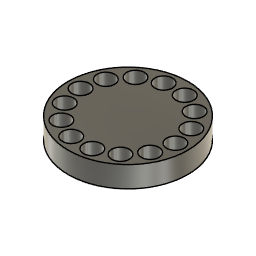
test_roller_pinion v1 (Autodesk Fusion 360 design; units mm, degrees)
Autodesk Fusion 360 part; units mm, degrees
note: some values were not read from the file. Chosen so that the rebuilt part matches the saved one: which face or edge a step refers to.
sketch "Sketch1" plane through (0, 0, 0) normal (0, 0, 1) x (1, 0, 0)
  circle A0 centre (0, 0) radius 17
  line L0 (-17, 0) -> (-16, 0)
  circle A1 centre (-13.5, 0) radius 2.5
  dimension "d1" = 34
  dimension "d2" = 5
  dimension "d7" = 1
  constraint coincident A0.centre origin
  constraint coincident A0 L0.start
  constraint horizontal L0
  constraint coincident L0.end A1
  measures "d1" diameter of A0
  measures "d2" diameter of A1
  measures "d7" distance of L0.start L0.end
extrude "Extrude1" add sketch "Sketch1" along normal blind 6
pattern_circular "C-Pattern1" count 14 over 360 about axis through (0, 0, 6) along (0, 0, 1) of 2 faces at (-15.9676, 0.401, 4) (-11.0081, -0.2012, 4)
sketch "Sketch2" plane through (0, 0, 6) normal (0, 0, 1) x (-1, 0, 0)
  circle A0 centre (-13.5, 0) radius 2.5
  circle A1 centre (-12.1631, 5.8574) radius 2.5
  circle A2 centre (-8.4171, 10.5547) radius 2.5
  circle A3 centre (-3.004, 13.1615) radius 2.5
  circle A4 centre (3.004, 13.1615) radius 2.5
  circle A5 centre (8.4171, 10.5547) radius 2.5
  circle A6 centre (12.1631, 5.8574) radius 2.5
  circle A7 centre (13.5, 0) radius 2.5
  circle A8 centre (0, 0) radius 17
  line L0 (11, 0) -> (16, 0)
  circle A9 centre (0, 0) radius 13.5
  circle A10 centre (12.1631, -5.8574) radius 2.5
  circle A11 centre (8.4171, -10.5547) radius 2.5
  circle A12 centre (3.004, -13.1615) radius 2.5
  circle A13 centre (-3.004, -13.1615) radius 2.5
  circle A14 centre (-8.4171, -10.5547) radius 2.5
  circle A15 centre (-12.1631, -5.8574) radius 2.5
  constraint coincident A7 L0.start
  constraint coincident A7 L0.end
  constraint horizontal L0
  constraint concentric A8 A9
  constraint coincident A7.centre A9
